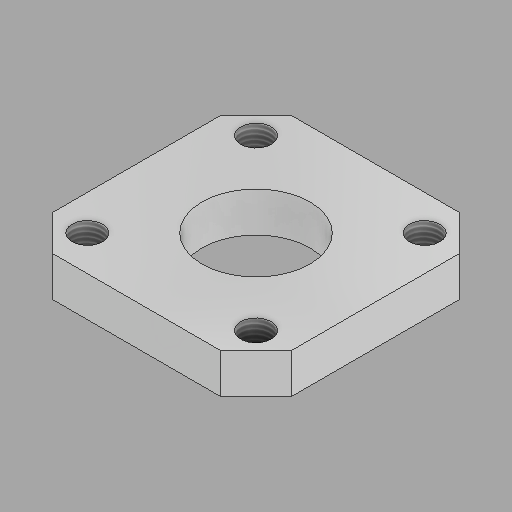
# Autodesk Inventor part: 00.32.004 "Flange"
Saved by Autodesk Inventor 2025.2 (Build 292293000, 293)
## iProperties
Created: 2024-12-06
Part Number: 00.32.004 "Flange"
Material: Steel
Document SubType Name: Modeling
Designer: Anna
Density: 7.85 g/cm^3
Appearance: Aluminum - Dark
Mass: 112.126 g
Surface Area: 255.114 cm^2
Volume: 112.126 cm^3
Author: Anna
Autodesk Inventor part; units mm, degrees
ref_plane "YZ Plane" through (0, 0, 0) normal (1, 0, 0) x (0, 1, 0)
ref_plane "XZ Plane" through (0, 0, 0) normal (0, 1, 0) x (-1, 0, 0)
ref_plane "XY Plane" through (0, 0, 0) normal (0, 0, 1) x (1, 0, 0)
sketch "Sketch1" plane through (0, 0, 0) normal (0, 1, 0) x (-1, 0, 0)
  line L0 (51, -51) -> (-51, -51)
  line L1 (-51, -51) -> (-51, 51)
  line L2 (-51, 51) -> (51, 51)
  line L3 (51, 51) -> (51, -51)
  line L4 (51, -51) -> (-51, 51) construction
  line L5 (-51, -51) -> (51, 51) construction
  point P0 (0, 0)
  dimension "d0" = 102
  dimension "d1" = 102
  constraints: 12 end point, 2 midpoint, 2 parallel, 1 horizontal, 1 perpendicular
  measures "d0" distance of L1.end L2.end
  measures "d1" distance of L0.end L1.end
extrude "Extrusion1" add sketch "Sketch1" along normal blind 17
chamfer "Chamfer1" distance 15 angle 45 4 edges at (51, 8.5, 51) (51, 8.5, -51) (-51, 8.5, -51) (-51, 8.5, 51)
sketch "Sketch2" plane through (0, 17, 0) normal (0, 1, 0) x (1, 0, 0)
  line L0 (51, -36) -> (51, 36) projected
  line L1 (-51, 36) -> (-51, -36) projected
  line L2 (51, -36) -> (36, -51) projected
  line L3 (36, 51) -> (-36, 51)
  circle A0 centre (36, -36) radius 6.5
  circle A1 centre (-36, -36) radius 6.5
  circle A2 centre (36, 36) radius 6.5
  circle A3 centre (-36, 36) radius 6.5
  circle A4 centre (0, 0) radius 23
  dimension "d7" = 13
  dimension "d8" = 13
  dimension "d9" = 13
  dimension "d10" = 13
  dimension "d22" = 46
  constraints: 5 centre point, 2 end point, 1 coincident
  measures "d7" diameter of A0
  measures "d8" diameter of A1
  measures "d9" diameter of A2
  measures "d10" diameter of A3
  measures "d22" diameter of A4
extrude "Extrusion2" cut sketch "Sketch2" against normal through all contours A0 | A1 | A2 | A3
thread "Thread1" size "M14x2" class "6H" standard "ANSI Metric M Profile" full length
thread "Thread2" size "M14x2" class "6H" standard "ANSI Metric M Profile" full length
thread "Thread3" size "M14x2" class "6H" standard "ANSI Metric M Profile" full length
thread "Thread4" size "M14x2" class "6H" standard "ANSI Metric M Profile" full length
sketch "Sketch3" plane through (0, 17, 0) normal (0, 1, 0) x (1, 0, 0)
  circle A0 centre (0, 0) radius 23
  dimension "d23" = 46
  constraints: 1 centre point, 1 coincident
  measures "d23" diameter of A0
extrude "Extrusion3" cut sketch "Sketch3" against normal through all
body "Solid1"
